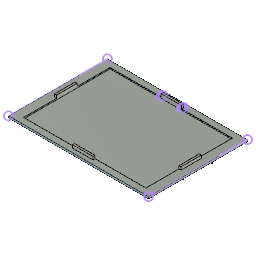
autopen_model_v1 (Autodesk Fusion 360 design; units mm, degrees)
part number: 2025-10-19-15-50-47-556
Autodesk Fusion 360 part; units mm, degrees
box "BoxPrimitive1" add length 240 width 327 height 5 placed x (0, 1, 0) y (-1, 0, 0) z (0, 0, 1) at (0, 0, 0)
cylinder "CylinderPrimitive1" add diameter 14 height 3 placed x (0, 1, 0) y (1, 0, 0) z (0, 0, -1) at (-15, 15, 0)
cylinder "CylinderPrimitive3" add diameter 14 height 5 placed x (0, 1, 0) y (1, 0, 0) z (0, 0, -1) at (-15, 225, 0)
cylinder "CylinderPrimitive4" add diameter 14 height 3 placed x (0, 1, 0) y (1, 0, 0) z (0, 0, -1) at (-312, 225, 0)
delete_face "DeleteFace1" 1 faces at (-21.6355, 222.7706, -1.6667)
cylinder "CylinderPrimitive5" add diameter 14 height 3 placed x (0, 1, 0) y (1, 0, 0) z (0, 0, -1) at (-15, 225, 0)
cylinder "CylinderPrimitive6" add diameter 14 height 3 placed x (0, 1, 0) y (1, 0, 0) z (0, 0, -1) at (-312, 15, 0)
sketch "Sketch8" plane through (0, 0, 5) normal (0, 0, 1) x (-1, 0, 0)
move_face "MoveFace1" by (-3, 0, 0) 1 faces at (-327, 160, 1.6667)
move_face "MoveFace2" by (-3, 0, 0) 2 faces at (-316.8388, 225.6005, -3) (-316.8388, 15.6005, -3)
move_face "MoveFace3" by (0, 0, -3) 2 faces at (-316.8388, 225.6005, -3) (-316.8388, 15.6005, -3)
delete_face "DeleteFace2" 1 faces at (-309.281, 231.4503, -2)
delete_face "DeleteFace3" 1 faces at (-309.6059, 8.4222, -2)
cylinder "CylinderPrimitive7" add diameter 14 height 3 placed x (0, 1, 0) y (1, 0, 0) z (0, 0, -1) at (-315, 225, 0)
cylinder "CylinderPrimitive8" add diameter 14 height 3 placed x (0, 1, 0) y (1, 0, 0) z (0, 0, -1) at (-315, 15, 0)
sketch "Sketch11" plane through (0, 0, 5) normal (0, 0, 1) x (-1, 0, 0)
  line L0 (0, -240) -> (330, -240)
  line L1 (330, -240) -> (330, 0)
  line L2 (330, 0) -> (0, 0)
  line L3 (0, 0) -> (0, -240)
  line L4 (190.7629, -15) -> (140.7629, -15)
  line L5 (140.7629, -15) -> (140.7629, -10)
  line L6 (140.7629, -10) -> (190.7629, -10)
  line L7 (190.7629, -10) -> (190.7629, -15)
  line L8 (140, -225) -> (190, -225)
  line L9 (190, -225) -> (190, -230)
  line L10 (190, -230) -> (140, -230)
  line L11 (140, -230) -> (140, -225)
  dimension "d35" = 330
  dimension "d47" = 15
  dimension "d48" = 15
  dimension "d49" = 240
  constraint perpendicular L4 L5
  constraint perpendicular L5 L6
  constraint perpendicular L4 L7
  constraint horizontal L8
  constraint vertical L9
  constraint horizontal L10
  constraint vertical L11
  measures "d35" distance of L0.start L0.end
  measures "d47" distance of L0 L8.end
  measures "d48" distance of L2 L4.start
  measures "d49" distance of L0.end L1.end
extrude "Extrude1" add sketch "Sketch11" along normal blind 7 contours L4 L5 L6 L7 | L8 L9 L10 L11
extrude "Extrude2" add 1 faces at (-330, 160, 1.6667) along direction (-1, 0, 0) blind 10
move_face "MoveFace4" by (-5, 0, 0) 1 faces at (-174.0962, 15, 7.3333)
move_face "MoveFace5" by (0, 5, 0) 1 faces at (-190.7629, 11.6667, 7.3333)
move_face "MoveFace6" by (5, 0, 0) 1 faces at (-174.0962, 13.3333, 12)
move_face "MoveFace7" by (-5, 0, 0) 5 faces at (-174.0962, 13.3333, 12) (-174.0962, 15, 7.3333) (-157.4295, 10, 7.3333) (-140.7629, 13.3333, 7.3333) (-190.7629, 11.6667, 7.3333)
move_face "MoveFace8" by (-5, 0, 0) 5 faces at (-156.6667, 226.6667, 12) (-173.3333, 225, 9.6667) (-190, 226.6667, 7.3333) (-140, 228.3333, 7.3333) (-173.3333, 230, 7.3333)
sketch "Sketch12" plane through (0, 0, 5) normal (0, 0, 1) x (-1, 0, 0)
  line L0 (145, -230) -> (145, -225)
  line L1 (195, -225) -> (195, -230)
  line L2 (0, -240) -> (340, -240)
  line L3 (340, -240) -> (340, 0)
  line L4 (340, 0) -> (0, 0)
  line L5 (0, 0) -> (0, -240)
  dimension "d56" = 145
  dimension "d57" = 145
  measures "d56" distance of L0.end L5
  measures "d57" distance of L1.start L3
sketch "Sketch13" plane through (0, 0, 5) normal (0, 0, 1) x (-1, 0, 0)
move_face "MoveFace9" by (0.763, 0, 0) 5 faces at (-162.4295, 10, 7.3333) (-162.4295, 11.6667, 12) (-162.4295, 15, 9.6667) (-145.7629, 13.3333, 7.3333) (-195.7629, 11.6667, 7.3333)
sketch "Sketch14" plane through (0, 0, 5) normal (0, 0, 1) x (-1, 0, 0)
  line L0 (340, -240) -> (340, 0)
  line L1 (0, 0) -> (0, -240)
sketch "Sketch15" plane through (0, 0, 5) normal (0, 0, 1) x (-1, 0, 0)
  line L0 (0, 0) -> (0, -240)
  line L1 (145, -225) -> (195, -225)
  line L2 (144.9999, -15) -> (194.9999, -15)
  line L3 (0, -240) -> (340, -240)
  line L4 (340, 0) -> (0, 0)
  line L5 (340, -240) -> (340, 0)
  line L6 (21.5, -170) -> (21.5, 0)
  line L7 (318.5, -225) -> (21.5, -225)
  line L8 (21.5, -225) -> (21.5, -15)
  line L9 (21.5, -15) -> (318.5, -15)
  line L10 (318.5, -15) -> (318.5, -225)
  line L11 (21.5, -145) -> (16.5, -145)
  line L12 (16.5, -145) -> (16.5, -95)
  line L13 (16.5, -95) -> (21.5, -95)
  line L14 (21.5, -95) -> (21.5, -145)
  line L15 (145, -230) -> (145, -225)
  line L16 (318.5, -145) -> (323.5, -145)
  line L17 (323.5, -145) -> (323.5, -95)
  line L18 (323.5, -95) -> (318.5, -95)
  line L19 (318.5, -95) -> (318.5, -145)
  point P0 (145, -225)
  point P1 (144.9999, -15)
  point P2 (195, -225)
  dimension "d69" = 15
  dimension "d70" = 15
  dimension "d81" = 5
  dimension "d82" = 240
  dimension "d86" = 5
  dimension "d87" = 297
  dimension "d88" = 210
  constraint coincident L4 L6.end
  constraint perpendicular L4 L6
  constraint horizontal L7
  constraint vertical L8
  constraint horizontal L9
  constraint vertical L10
  constraint coincident L6 L8.end
  constraint horizontal L11
  constraint vertical L12
  constraint horizontal L13
  constraint vertical L14
  constraint coincident L6 L11.start
  constraint horizontal L16
  constraint vertical L17
  constraint horizontal L18
  constraint vertical L19
  constraint coincident L10 L16.start
  measures "d69" distance of P2 L3
  measures "d70" distance of L2.end L4
  measures "d81" distance of P0 L15.start
  measures "d82" distance of L0.start L0.end
  measures "d86" distance of L16.start L16.end
  measures "d87" distance of L11.start L16.start
  measures "d88" vertical distance of P0 P1
extrude "Extrude3" add sketch "Sketch15" along normal blind 7 contours L10 L16 L17 L18 L19 | L6 L8 L11 L12 L13 L14
sketch "Sketch16" plane through (0, 0, 5) normal (0, 0, 1) x (-1, 0, 0)
  line L0 (21.5, -225) -> (318.5, -225)
  line L1 (318.5, -225) -> (318.5, -15)
  line L2 (318.5, -15) -> (21.5, -15)
  line L3 (21.5, -15) -> (21.5, -225)
  constraint horizontal L0
  constraint vertical L1
  constraint horizontal L2
  constraint vertical L3
extrude "Extrude4" cut sketch "Sketch16" against normal blind 3
sketch "Sketch17" plane through (0, 0, 0) normal (0, -1, 0) x (1, 0, 0)
  line L0 (-340, 0) -> (0, 0)
  line L1 (0, 0) -> (0, 5)
  line L2 (0, 5) -> (-340, 5)
  line L3 (-340, 5) -> (-340, 0)
sketch "Sketch18" plane through (0, 0, 5) normal (0, 0, 1) x (-1, 0, 0)
sketch "Sketch19" plane through (0, 0, 5) normal (0, 0, 1) x (-1, 0, 0)
sketch "Sketch20" plane through (0, 0, 0) normal (0, 0, -1) x (1, 0, 0)
  circle A0 centre (-15, -225) radius 7
  circle A1 centre (-15, -15) radius 7
  line L0 (-340, -240) -> (0, -240)
  line L1 (0, -240) -> (0, 0)
  line L2 (0, 0) -> (-340, 0)
  line L3 (-340, 0) -> (-340, -240)
sketch "Sketch21" plane through (0, 0, 0) normal (0, 0, -1) x (1, 0, 0)
  line L0 (-15, -156) -> (0, -156)
  line L1 (-15, -86) -> (0, -86)
  line L2 (-15, -86) -> (-340, -86)
  line L3 (-15, -156) -> (-340, -156)
  line L4 (-15, -154) -> (0, -154)
  line L5 (-15, -154) -> (-340, -154)
  line L6 (-15, -84) -> (-340, -84)
  line L7 (-15, -84) -> (0, -84)
  line L8 (0, -156) -> (-340, -156)
  line L9 (-340, -156) -> (-340, -154)
  line L10 (-340, -154) -> (0, -154)
  line L11 (0, -154) -> (0, -156)
  line L12 (-340, -86) -> (0, -86)
  line L13 (0, -86) -> (0, -84)
  line L14 (0, -84) -> (-340, -84)
  line L15 (-340, -84) -> (-340, -86)
  constraint horizontal L8
  constraint vertical L9
  constraint horizontal L10
  constraint vertical L11
  constraint horizontal L12
  constraint vertical L13
  constraint horizontal L14
  constraint vertical L15
extrude "Extrude5" add sketch "Sketch21" along normal blind 3
move_face "MoveFace10" to x (1, 0, 0) y (0, 1, 0) z (0, 0, 1) at (-8, 0, 0) 2 faces at (-319.8388, 15.6005, -3) (-312.6059, 8.4222, -1)
move_face "MoveFace11" to x (1, 0, 0) y (0, 1, 0) z (0, 0, 1) at (-8, 0, 0) 2 faces at (-319.8388, 225.6005, -3) (-312.281, 231.4503, -1)
